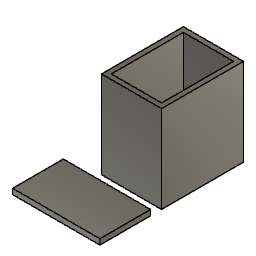
boks v1 (Autodesk Fusion 360 design; units mm, degrees)
Autodesk Fusion 360 part; units mm, degrees
box "BoxPrimitive1" add length 150 width 110 height 160 placed x (0, 1, 0) y (-1, 0, 0) z (0, 0, 1) at (110, 0, 0) makes body 1
shell "Shell1" thickness 9 removed faces 1 at (36.6667, 50, 160) on bodies 1
box "BoxPrimitive3" add length 92.9707 width 160 height 10 placed x (0, -1, 0) y (1, 0, 0) z (0, 0, 1) at (-50, -20, 0) separate body makes body 2
shell "Shell2" thickness 8 removed faces 1 at (56.6667, -50.9902, 0) on bodies 2
